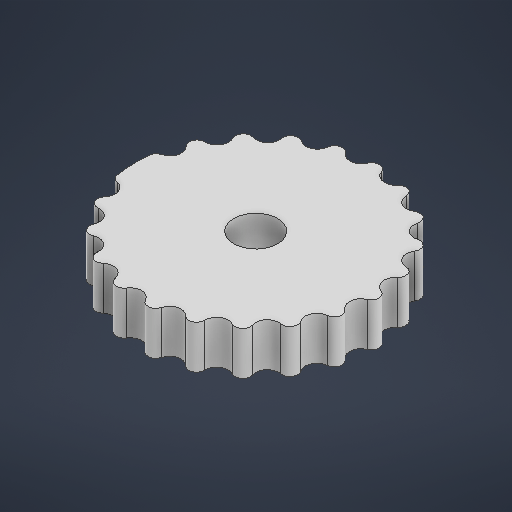
# Autodesk Inventor part: RuedaDentada
Saved by Autodesk Inventor 2026.1 (Build 301233020, 233B)
## iProperties
Created: 2025-10-19
Part Number: RuedaDentada
Material: Generic
Document SubType Name: Modeling
Designer: tito.luyo
Density: 1 g/cm^3
Appearance: Default
Author: tito.luyo
Autodesk Inventor part; units mm, degrees
ref_plane "YZ Plane" through (0, 0, 0) normal (1, 0, 0) x (0, 1, 0)
ref_plane "XZ Plane" through (0, 0, 0) normal (0, 1, 0) x (-1, 0, 0)
ref_plane "XY Plane" through (0, 0, 0) normal (0, 0, 1) x (1, 0, 0)
sketch "Sketch1" plane through (0, 0, 0) normal (0, 1, 0) x (-1, 0, 0)
  line L0 (0, 0) -> (45.711006, 0) construction
  line L1 (45.711006, 0) -> (45.711006, -43.57398) construction
  line L2 (45.711006, -43.57398) -> (0, -43.57398) construction
  line L3 (0, -43.57398) -> (0, 0) construction
  circle A0 centre (22.564458, -20.680957) radius 19.33557
  line L4 (25.344393, -20.680957) -> (41.900028, -20.680957)
  line L5 (22.564458, -20.680957) -> (39.120092, -20.680957) construction
  circle A1 centre (40.970521, -14.522375) radius 1.85
  line L6 (22.564458, -20.680957) -> (40.970521, -14.522375) construction
  line L7 (0, 0) -> (60, 0)
  line L8 (60, 0) -> (60, -60)
  line L9 (60, -60) -> (0, -60)
  line L10 (0, -60) -> (0, 0)
  circle A2 centre (38.678727, -12.434869) radius 1.25
  circle A3 centre (38.326229, -9.354976) radius 1.85
  line L11 (22.564458, -20.680957) -> (38.326229, -9.354976) construction
  circle A4 centre (35.519636, -8.038529) radius 1.25
  circle A5 centre (34.272153, -5.200609) radius 1.85
  line L12 (22.564458, -20.680957) -> (34.272153, -5.200609) construction
  circle A6 centre (31.201791, -4.772969) radius 1.25
  circle A7 centre (26.111395, -2.930271) radius 1.25
  line L13 (22.564458, -20.680957) -> (29.170902, -2.430856) construction
  circle A8 centre (29.170902, -2.430856) radius 1.85
  circle A9 centre (23.478749, -1.293452) radius 1.85
  line L14 (22.564458, -20.680957) -> (23.478749, -1.293452) construction
  circle A10 centre (20.703749, -2.675253) radius 1.25
  circle A11 centre (15.462532, -4.030724) radius 1.25
  line L15 (22.564458, -20.680957) -> (17.704819, -1.890129) construction
  circle A12 centre (17.704819, -1.890129) radius 1.85
  line L16 (22.564458, -20.680957) -> (12.365551, -4.16752) construction
  circle A13 centre (10.856533, -6.875447) radius 1.25
  circle A14 centre (12.365551, -4.16752) radius 1.85
  circle A15 centre (4.819655, -12.817543) radius 1.85
  line L17 (22.564458, -20.680957) -> (4.819655, -12.817543) construction
  circle A16 centre (5.104433, -15.904435) radius 1.25
  circle A17 centre (4.472818, -21.281119) radius 1.25
  line L18 (22.564458, -20.680957) -> (3.287957, -18.416489) construction
  circle A18 centre (3.287957, -18.416489) radius 1.85
  circle A19 centre (7.975873, -31.397338) radius 1.25
  circle A20 centre (5.379807, -29.703101) radius 1.85
  line L19 (22.564458, -20.680957) -> (5.379807, -29.703101) construction
  line L20 (22.564458, -20.680957) -> (3.480412, -24.217976) construction
  circle A21 centre (5.459378, -26.604122) radius 1.25
  circle A22 centre (3.480412, -24.217976) radius 1.85
  circle A23 centre (21.901148, -38.770392) radius 1.25
  circle A24 centre (18.960845, -39.75254) radius 1.85
  circle A25 centre (16.581621, -37.765257) radius 1.25
  circle A26 centre (13.482384, -37.83401) radius 1.85
  circle A27 centre (11.797219, -35.232046) radius 1.25
  circle A28 centre (8.816253, -34.381255) radius 1.85
  line L21 (22.564458, -20.680957) -> (8.816253, -34.381255) construction
  line L22 (22.564458, -20.680957) -> (13.482384, -37.83401) construction
  line L23 (22.564458, -20.680957) -> (18.960845, -39.75254) construction
  circle A29 centre (30.365883, -38.4531) radius 1.85
  circle A30 centre (24.761625, -39.965245) radius 1.85
  circle A31 centre (27.280004, -38.157549) radius 1.25
  circle A32 centre (32.237086, -35.981542) radius 1.25
  line L24 (22.564458, -20.680957) -> (30.365883, -38.4531) construction
  line L25 (22.564458, -20.680957) -> (24.761625, -39.965245) construction
  circle A33 centre (35.272356, -35.351357) radius 1.85
  circle A34 centre (36.329016, -32.437001) radius 1.25
  line L26 (22.564458, -20.680957) -> (35.272356, -35.351357) construction
  circle A35 centre (40.563557, -22.604506) radius 1.25
  circle A36 centre (41.338208, -25.606158) radius 1.85
  line L27 (22.564458, -20.680957) -> (41.338208, -25.606158) construction
  circle A37 centre (39.189799, -27.840961) radius 1.25
  circle A38 centre (39.042194, -30.937444) radius 1.85
  line L28 (22.564458, -20.680957) -> (39.042194, -30.937444) construction
  circle A39 centre (40.396505, -17.568767) radius 1.25
  circle A40 centre (7.29773, -10.954979) radius 1.25
  circle A41 centre (7.938507, -7.921927) radius 1.85
  line L29 (22.564458, -20.680957) -> (7.938507, -7.921927) construction
  circle A42 centre (22.564458, -20.680957) radius 3.55
  point P0 (40.875917, -23.81485)
  point P1 (41.767546, -22.94053)
  point P2 (41.646473, -17.55991)
  point P3 (40.627963, -16.340383)
  point P4 (39.602837, -13.276605)
  point P5 (38.536591, -11.192977)
  point P6 (36.651327, -8.569354)
  point P7 (35.016618, -6.894207)
  point P8 (32.43984, -4.945404)
  point P9 (30.382884, -3.828568)
  point P10 (27.345067, -2.728894)
  point P11 (25.049844, -2.270263)
  point P12 (21.822701, -2.118075)
  point P13 (19.494503, -2.358671)
  point P14 (16.36668, -3.167581)
  point P15 (14.213749, -4.085884)
  point P16 (11.465008, -5.783541)
  point P17 (9.67991, -7.297414)
  point P18 (7.556108, -9.731974)
  point P19 (6.298506, -11.706013)
  point P20 (4.989603, -14.659721)
  point P21 (4.371983, -16.91736)
  point P22 (3.995052, -20.126026)
  point P23 (4.072654, -22.465335)
  point P24 (4.661408, -25.641966)
  point P25 (5.427293, -27.85371)
  point P26 (6.929072, -30.714178)
  point P27 (8.314736, -32.600531)
  point P28 (10.595216, -34.888985)
  point P29 (12.476721, -36.281225)
  point P30 (15.331929, -37.79298)
  point P31 (17.540986, -38.566581)
  point P32 (20.715542, -39.166419)
  point P33 (23.054566, -39.252188)
  point P34 (26.264529, -38.886459)
  point P35 (28.52431, -38.276723)
  point P36 (31.482569, -36.978138)
  point P37 (33.460985, -35.727435)
  point P38 (35.902944, -33.612144)
  point P39 (37.423039, -31.832341)
  point P40 (39.130281, -29.089543)
  point P41 (40.056093, -26.939831)
  point P42 (32.721601, -37.13382)
  point P43 (33.070154, -36.913474)
  dimension "d39" = 0
  dimension "circ_mayor" = 3.7
  dimension "d126" = 19.40905
  dimension "d132" = 18.5
  dimension "d133" = 60
  dimension "d134" = 60
  dimension "pos_circ_y" = 22.56446
  dimension "pos_circ_x" = 20.68096
  dimension "circ_menor" = 2.5
  dimension "d157" = 3.7
  dimension "d158" = 19.40905
  dimension "d160" = 2.5
  dimension "d166" = 17.2
  dimension "d167" = 3.7
  dimension "d168" = 19.40905
  dimension "d169" = 2.5
  dimension "d170" = 3.7
  dimension "d171" = 19.40905
  dimension "d172" = 2.5
  dimension "d173" = 17.2
  dimension "d177" = 17.2
  dimension "d178" = 3.7
  dimension "d179" = 19.40905
  dimension "d180" = 2.5
  dimension "d181" = 3.7
  dimension "d182" = 19.40905
  dimension "d183" = 2.5
  dimension "d184" = 17.2
  dimension "d185" = 3.7
  dimension "d186" = 19.40905
  dimension "d187" = 2.5
  dimension "d192" = 17.2
  dimension "d196" = 17.2
  dimension "d197" = 3.7
  dimension "d198" = 19.40905
  dimension "d199" = 2.5
  dimension "d200" = 3.7
  dimension "d201" = 19.40905
  dimension "d202" = 2.5
  dimension "d203" = 17.2
  dimension "d204" = 3.7
  dimension "d205" = 19.40905
  dimension "d206" = 2.5
  dimension "d207" = 3.7
  dimension "d208" = 19.40905
  dimension "d209" = 2.5
  dimension "d210" = 17.2
  dimension "d211" = 17.2
  dimension "d212" = 3.7
  dimension "d213" = 19.40905
  dimension "d214" = 2.5
  dimension "d215" = 3.7
  dimension "d216" = 19.40905
  dimension "d217" = 2.5
  dimension "d218" = 17.2
  dimension "d219" = 3.7
  dimension "d220" = 19.40905
  dimension "d221" = 2.5
  dimension "d226" = 17.2
  dimension "d227" = 17.2
  dimension "d253" = 3.7
  dimension "d254" = 19.40905
  dimension "d255" = 2.5
  dimension "d256" = 3.7
  constraints: 52 end point, 42 centre point, 20 tangent, 2 coincident, 2 horizontal, 2 parallel, 1 collinear, 1 perpendicular, 5 other
  measures "d39" distance between parallel lines of L4 L5
  measures "circ_mayor" diameter of A1
  measures "d126" distance of L5.start L6.end
  measures "d132" angle of L4 L6
  measures "d133" distance of L8.end L9.end
  measures "d134" distance of L7.end L8.end
  measures "pos_circ_y" distance from line of L10 point (22.564, -20.681)
  measures "pos_circ_x" distance from line of L7 point (22.564, -20.681)
  measures "circ_menor" diameter of A2
  measures "d157" diameter of A3
  measures "d158" distance of L5.start L11.end
  measures "d160" diameter of A4
  measures "d166" angle of L6 L11
  measures "d167" diameter of A5
  measures "d168" distance of L5.start L12.end
  measures "d169" diameter of A6
  measures "d170" diameter of A8
  measures "d171" distance of L5.start L13.end
  measures "d172" diameter of A7
  measures "d173" angle of L12 L13
  measures "d177" angle of L11 L12
  measures "d178" diameter of A9
  measures "d179" distance of L5.start L14.end
  measures "d180" diameter of A10
  measures "d181" diameter of A12
  measures "d182" distance of L5.start L15.end
  measures "d183" diameter of A11
  measures "d184" angle of L14 L15
  measures "d185" diameter of A14
  measures "d186" distance of L5.start L16.end
  measures "d187" diameter of A13
  measures "d192" angle of L15 L16
  measures "d196" angle of L13 L14
  measures "d197" diameter of A15
  measures "d198" distance of L23.start L17.end
  measures "d199" diameter of A16
  measures "d200" diameter of A18
  measures "d201" distance of L23.start L18.end
  measures "d202" diameter of A17
  measures "d203" angle of L17 L18
  measures "d204" diameter of A22
  measures "d205" distance of L23.start L20.end
  measures "d206" diameter of A21
  measures "d207" diameter of A20
  measures "d208" distance of L23.start L19.end
  measures "d209" diameter of A19
  measures "d210" angle of L20 L19
  measures "d211" angle of L18 L20
  measures "d212" diameter of A28
  measures "d213" distance of L23.start L21.end
  measures "d214" diameter of A27
  measures "d215" diameter of A26
  measures "d216" distance of L23.start L22.end
  measures "d217" diameter of A25
  measures "d218" angle of L21 L22
  measures "d219" diameter of A24
  measures "d220" distance of L23.start L23.end
  measures "d221" diameter of A23
  measures "d226" angle of L22 L23
  measures "d227" angle of L19 L21
  measures "d253" diameter of A30
  measures "d254" distance of L24.start L25.end
  measures "d255" diameter of A31
  measures "d256" diameter of A29
sketch "Sketch1 outline for Extrusion1" plane through (0, 0, 0) normal (0, 1, 0) x (-1, 0, 0)
  arc A0 (33.070154, -36.913474) -> (33.460985, -35.727435) centre (32.237086, -35.981542) ccw
  arc A1 (33.460985, -35.727435) -> (35.902944, -33.612144) centre (35.272356, -35.351357) cw
  arc A2 (35.902944, -33.612144) -> (37.423039, -31.832341) centre (36.329016, -32.437001) ccw
  arc A3 (37.423039, -31.832341) -> (39.130281, -29.089543) centre (39.042194, -30.937444) cw
  arc A4 (39.130281, -29.089543) -> (40.056093, -26.939831) centre (39.189799, -27.840961) ccw
  arc A5 (40.056093, -26.939831) -> (40.875917, -23.81485) centre (41.338208, -25.606158) cw
  arc A6 (40.875917, -23.81485) -> (41.767546, -22.94053) centre (40.563557, -22.604506) ccw
  arc A7 (41.767546, -22.94053) -> (41.646473, -17.55991) centre (22.564458, -20.680957) ccw
  arc A8 (41.646473, -17.55991) -> (40.627963, -16.340383) centre (40.396505, -17.568767) ccw
  arc A9 (40.627963, -16.340383) -> (39.602837, -13.276605) centre (40.970521, -14.522375) cw
  arc A10 (39.602837, -13.276605) -> (38.536591, -11.192977) centre (38.678727, -12.434869) ccw
  arc A11 (38.536591, -11.192977) -> (36.651327, -8.569354) centre (38.326229, -9.354976) cw
  arc A12 (36.651327, -8.569354) -> (35.016618, -6.894207) centre (35.519636, -8.038529) ccw
  arc A13 (35.016618, -6.894207) -> (32.43984, -4.945404) centre (34.272153, -5.200609) cw
  arc A14 (32.43984, -4.945404) -> (30.382884, -3.828568) centre (31.201791, -4.772969) ccw
  arc A15 (30.382884, -3.828568) -> (27.345067, -2.728894) centre (29.170902, -2.430856) cw
  arc A16 (27.345067, -2.728894) -> (25.049844, -2.270263) centre (26.111395, -2.930271) ccw
  arc A17 (25.049844, -2.270263) -> (21.822701, -2.118075) centre (23.478749, -1.293452) cw
  arc A18 (21.822701, -2.118075) -> (19.494503, -2.358671) centre (20.703749, -2.675253) ccw
  arc A19 (19.494503, -2.358671) -> (16.36668, -3.167581) centre (17.704819, -1.890129) cw
  arc A20 (16.36668, -3.167581) -> (14.213749, -4.085884) centre (15.462532, -4.030724) ccw
  arc A21 (14.213749, -4.085884) -> (11.465008, -5.783541) centre (12.365551, -4.16752) cw
  arc A22 (11.465008, -5.783541) -> (9.67991, -7.297414) centre (10.856533, -6.875447) ccw
  arc A23 (9.67991, -7.297414) -> (7.556108, -9.731974) centre (7.938507, -7.921927) cw
  arc A24 (7.556108, -9.731974) -> (6.298506, -11.706013) centre (7.29773, -10.954979) ccw
  arc A25 (6.298506, -11.706013) -> (4.989603, -14.659721) centre (4.819655, -12.817543) cw
  arc A26 (4.989603, -14.659721) -> (4.371983, -16.91736) centre (5.104433, -15.904435) ccw
  arc A27 (4.371983, -16.91736) -> (3.995052, -20.126026) centre (3.287957, -18.416489) cw
  arc A28 (3.995052, -20.126026) -> (4.072654, -22.465335) centre (4.472818, -21.281119) ccw
  arc A29 (4.072654, -22.465335) -> (4.661408, -25.641966) centre (3.480412, -24.217976) cw
  arc A30 (4.661408, -25.641966) -> (5.427293, -27.85371) centre (5.459378, -26.604122) ccw
  arc A31 (5.427293, -27.85371) -> (6.929072, -30.714178) centre (5.379807, -29.703101) cw
  arc A32 (6.929072, -30.714178) -> (8.314736, -32.600531) centre (7.975873, -31.397338) ccw
  arc A33 (8.314736, -32.600531) -> (10.595216, -34.888985) centre (8.816253, -34.381255) cw
  arc A34 (10.595216, -34.888985) -> (12.476721, -36.281225) centre (11.797219, -35.232046) ccw
  arc A35 (12.476721, -36.281225) -> (15.331929, -37.79298) centre (13.482384, -37.83401) cw
  arc A36 (15.331929, -37.79298) -> (17.540986, -38.566581) centre (16.581621, -37.765257) ccw
  arc A37 (17.540986, -38.566581) -> (20.715542, -39.166419) centre (18.960845, -39.75254) cw
  arc A38 (20.715542, -39.166419) -> (23.054566, -39.252188) centre (21.901148, -38.770392) ccw
  arc A39 (23.054566, -39.252188) -> (26.264529, -38.886459) centre (24.761625, -39.965245) cw
  arc A40 (26.264529, -38.886459) -> (28.52431, -38.276723) centre (27.280004, -38.157549) ccw
  arc A41 (28.52431, -38.276723) -> (31.482569, -36.978138) centre (30.365883, -38.4531) cw
  arc A42 (31.482569, -36.978138) -> (32.721601, -37.13382) centre (32.237086, -35.981542) ccw
  arc A43 (32.721601, -37.13382) -> (33.070154, -36.913474) centre (22.564458, -20.680957) ccw
  circle A44 centre (22.564458, -20.680957) radius 3.55
extrude "Extrusion1" add sketch "Sketch1 outline for Extrusion1" along normal blind 7
equation "\"angulo\" = 17.2deg"
equation "\"sep\" = 19.40905"
equation "\"d144\" = 19.40905"
equation "\"d148\" = 19.40905"
equation "\"d162\" = 19.40905"
equation "\"d163\" = 19.40905"
equation "\"d164\" = 17.2deg"
equation "\"d174\" = 19.40905"
equation "\"d175\" = 17.2deg"
equation "\"d193\" = 19.40905"
equation "\"d194\" = 17.2deg"
equation "\"d228\" = 19.40905"
equation "\"d229\" = 17.2deg"
equation "\"d247\" = 19.40905"
equation "\"d250\" = 17.2deg"
equation "\"d261\" = 19.40905"
equation "\"d263\" = 17.2deg"
equation "\"d278\" = 19.40905"
equation "\"d280\" = 17.2deg"
equation "\"d281\" = 17.2deg"
equation "\"d289\" = 19.40905"
body "Solid1"
